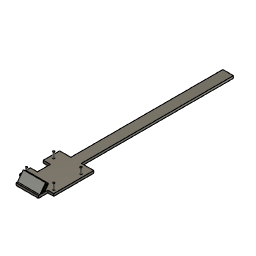
HUD_mount_v3 (Autodesk Fusion 360 design; units mm, degrees)
Autodesk Fusion 360 part; units mm, degrees
sketch "Sketch1" plane through (0, 0, 0) normal (0, 1, 0) x (1, 0, 0)
  line L0 (-10, -121.4) -> (10, -121.4)
  line L1 (0, -121.4) -> (0, -135.9)
  line L2 (14.5, -121.4) -> (-14.5, -121.4)
  line L3 (-14.5, -121.4) -> (-14.5, -150.4)
  line L4 (-14.5, -150.4) -> (14.5, -150.4)
  line L5 (14.5, -150.4) -> (14.5, -121.4)
  line L6 (14.5, -121.4) -> (-14.5, -150.4) construction
  line L7 (-14.5, -121.4) -> (14.5, -150.4) construction
  line L8 (13.65, -122.25) -> (-13.65, -122.25)
  line L9 (-13.65, -122.25) -> (-13.65, -149.55)
  line L10 (-13.65, -149.55) -> (13.65, -149.55)
  line L11 (13.65, -149.55) -> (13.65, -122.25)
  line L12 (13.65, -122.25) -> (-13.65, -149.55) construction
  line L13 (-13.65, -122.25) -> (13.65, -149.55) construction
  line L14 (-13.65, -124.3) -> (-11.6, -124.3)
  line L15 (-11.6, -124.3) -> (11.6, -124.3)
  line L16 (11.6, -124.3) -> (11.6, -147.5)
  line L17 (11.6, -147.5) -> (-11.6, -147.5)
  line L18 (-11.6, -147.5) -> (-11.6, -124.3)
  line L19 (-11.6, -124.3) -> (11.6, -147.5) construction
  line L20 (11.6, -124.3) -> (-11.6, -147.5) construction
  circle A0 centre (-11.6, -124.3) radius 0.75
  circle A1 centre (11.6, -124.3) radius 0.75
  circle A2 centre (-11.6, -147.5) radius 0.75
  circle A3 centre (11.6, -147.5) radius 0.75
  line L21 (0, -135.9) -> (9.63, -135.9)
  line L22 (9.63, -135.9) -> (9.63, -113)
  line L23 (-14.5, -121.4) -> (-14.5, -41.4)
  line L24 (14.5, -121.4) -> (14.5, -41.4)
  line L25 (-14.5, -41.4) -> (14.5, -41.4)
  line L26 (9.63, -135.9) -> (-9.63, -135.9)
  line L27 (-9.63, -135.9) -> (-9.63, -113)
  line L28 (-9.63, -135.9) -> (-9.63, -150.4)
  line L29 (9.63, -135.9) -> (9.63, -150.4)
  line L30 (-14.5, -116.3321) -> (-5, -116.3321)
  line L31 (-5, -116.3321) -> (-5, 13)
  line L32 (-5, 13) -> (4, 13)
  line L33 (4, 13) -> (4, -116.3321)
  line L34 (4, -116.3321) -> (14.5, -116.3321)
  line L35 (-14.5, -116.3321) -> (-14.5, -130.3321)
  line L36 (-14.5, -130.3321) -> (-8.5, -130.3321)
  line L37 (-8.5, -130.3321) -> (-8.5, -141.3321)
  line L38 (-8.5, -141.3321) -> (-14.5, -141.3321)
  point P0 (0, -135.9)
  point P1 (0, -135.9)
  point P2 (0, -135.9)
  dimension "d22" = 14.5
  dimension "d23" = 29
  dimension "d24" = 29
  dimension "d25" = 27.3
  dimension "d26" = 27.3
  dimension "d35" = 2.05
  dimension "d36" = 1.5
  dimension "d37" = 1.5
  dimension "d38" = 1.5
  dimension "d39" = 1.5
  dimension "d40" = 9.63
  dimension "d41" = 80
  dimension "d42" = 80
  dimension "d43" = 19.26
  dimension "d59" = 14
  dimension "d60" = 6
  dimension "d61" = 11
  constraint midpoint L0 L1.start
  constraint perpendicular L0 L1
  constraint horizontal L2
  constraint perpendicular L2 L3
  constraint parallel L2 L4
  constraint parallel L3 L5
  constraint coincident L6 P2
  constraint coincident L7 P2
  constraint coincident P2 P1
  constraint horizontal L8
  constraint perpendicular L8 L9
  constraint parallel L8 L10
  constraint parallel L9 L11
  constraint coincident L12 P2
  constraint coincident L13 P2
  constraint coincident L9 L14.start
  constraint perpendicular L9 L14
  constraint horizontal L15
  constraint perpendicular L15 L16
  constraint parallel L15 L17
  constraint parallel L16 L18
  constraint coincident L19 P2
  constraint coincident L20 P2
  constraint coincident L14.end L15.start
  constraint coincident L15.end L16.start
  constraint coincident L17.end L18.start
  constraint coincident L16.end L17.start
  constraint horizontal L21
  constraint perpendicular L21 L22
  constraint perpendicular L2 L23
  constraint perpendicular L2 L24
  constraint perpendicular L22 L26
  constraint perpendicular L15 L27
  constraint coincident L4 L28.end
  constraint perpendicular L4 L28
  constraint coincident L4 L29.end
  constraint perpendicular L4 L29
  constraint coincident L23 L30.start
  constraint perpendicular L23 L30
  constraint perpendicular L30 L31
  constraint perpendicular L31 L32
  constraint perpendicular L30 L33
  constraint coincident L24 L34.end
  constraint perpendicular L24 L34
  constraint perpendicular L30 L35
  constraint perpendicular L18 L36
  constraint perpendicular L36 L37
  constraint coincident L3 L38.end
  constraint perpendicular L3 L38
  measures "d22" distance of L1.start P2
  measures "d23" distance of L3.end L4.end
  measures "d24" distance of L2.end L3.end
  measures "d25" distance of L9.end L10.end
  measures "d26" distance of L8.end L9.end
  measures "d35" distance of L14.start L14.end
  measures "d36" diameter of A0
  measures "d37" diameter of A1
  measures "d38" diameter of A2
  measures "d39" diameter of A3
  measures "d40" distance of P2 L21.end
  measures "d41" distance of L2.end L23.end
  measures "d42" distance of L2.start L24.end
  measures "d43" distance of L21.end L26.end
  measures "d59" distance of L30.start L35.end
  measures "d60" distance of L35.end L36.end
  measures "d61" distance of L36.end L37.end
extrude "Extrude6" add sketch "Sketch1" along normal blind 2 contours L0 L2 L23 L27 L30 L35 | L0 L2 L3 L8 L9 L27 L35 L36 | L0 L2 L22 L25 L27 L30 L31 L33 L34 | L0 L1 L2 L8 L27 | L0 L1 L2 L8 L22 | L8 L9 L14 L15 A0 L27 | L1 L8 L15 L27 | L0 L2 L22 L24 L34 | L0 L2 L4 L5 L8 L10 L11 L22 L29 | L1 L8 L15 L22 | L15 L18 A0 L27 L36 | L1 L15 L26 L27 L36 L37 | L3 L4 L9 L10 L28 L38 | L9 L14 L18 A0 L36 | L8 L10 L11 L15 L16 L17 A1 A3 L22 L29 | L1 L15 L21 L22 L26 | L15 L18 A0 | L14 L15 A0 | L25 L31 L32 L33 | L9 L10 L17 L18 A2 L28 L38 | L15 L16 L17 A1 A3 L22 L29 | L17 L21 L26 L28 L29 L37 L38 | L14 L18 A0 | L4 L10 L28 L29 | L17 L18 A2 L28 L38 | L15 L16 A1 | L15 L16 A1 | L10 L17 L28 L29 | L17 L18 A2 | L17 L18 A2 | L16 L17 A3 | L16 L17 A3 makes body 1
combine "Combine1" [no effect]
extrude "Extrude7" add sketch "Sketch1" along normal blind 7 separate body contours L15 L18 A0 | L14 L15 A0 | L14 L18 A0 | L15 L16 A1 | L15 L16 A1 | L17 L18 A2 | L17 L18 A2 | L16 L17 A3 | L16 L17 A3 makes body 2 at (-12.1978, 2.3333, 123.8471) makes body 3 at (12.2587, 2.3333, 147.1413) makes body 4 at (-10.9089, 4.6667, 147.2087) makes body 5 at (11.1037, 2.3333, 124.8623)
sketch "Sketch3" plane through (14.5, 0, 0) normal (1, 0, 0) x (0, 0, -1)
  line L0 (-150.4, 2, -14.5) -> (-158.4, 2, -14.5)
  line L1 (-158.4, 2, -14.5) -> (-158.4, 0, -14.5)
  line L2 (-158.4, 0, -14.5) -> (-150.4, 0, -14.5)
  line L3 (-158.4, 2, -14.5) -> (-157.2, 2, -14.5)
  line L4 (-152.2831, 8.5249, -14.5) -> (-151.4845, 7.9231, -14.5)
  line L5 (-151.4845, 7.9231, -14.5) -> (-155.9479, 2, -14.5)
  line L6 (-151.4845, 7.9231, -14.5) -> (-150.606, 7.2611, -14.5)
  line L7 (-150.606, 7.2611, -14.5) -> (-149.8074, 6.6593, -14.5)
  line L8 (-149.8074, 6.6593, -14.5) -> (-153.3184, 2, -14.5)
  line L9 (-150.606, 7.2611, -14.5) -> (-154.5705, 2, -14.5)
  line L10 (-152.2831, 8.5249, -14.5) -> (-157.2, 2, -14.5)
  line L11 (-150.4, 2, -14.5) -> (-150.4, 0, -14.5)
  dimension "d66" = 8
  dimension "d67" = 1.2
  dimension "d69" = 1
  dimension "d70" = 1.1
  dimension "d71" = 1
extrude "Extrude8" add sketch "Sketch3" along normal blind 9.5 contours L0 L1 L2 L3 L11 | L0 L7 L8 L9 | L0 L4 L5 L10 in plane through (0, 0, 0) normal (1, 0, 0) bodies 1
move_face "OffsetFaces1" offset 9.5 1 faces at (0, 0.6667, 154.4568) on bodies 1
combine "Combine2" operation add target body 2 tool bodies 3 1 5 4
equation "d22 = ( 29 / 2 ) * 1 mm"
equation "d40 = ( 19.26 / 2 ) * 1 mm"
